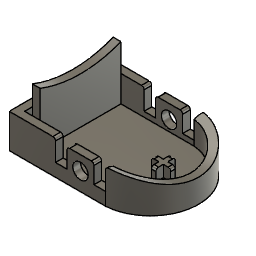
Vacuum_release_button (Autodesk Fusion 360 design; units mm, degrees)
Autodesk Fusion 360 part; units mm, degrees
sketch "Sketch1" plane through (0, 0, 0) normal (0, 1, 0) x (1, 0, 0)
  line L0 (-13.97, -9.525) -> (-13.97, 9.525)
  line L1 (-13.97, 9.525) -> (13.97, 9.525)
  line L2 (13.97, 9.525) -> (13.97, -9.525)
  line L3 (13.97, -9.525) -> (-13.97, 9.525) construction
  line L4 (-13.97, -9.525) -> (13.97, 9.525) construction
  line L5 (5.08, 9.525) -> (5.08, -9.525) construction
  line L6 (5.08, 0) -> (13.97, 0) construction
  arc A0 (5.08, -9.525) -> (5.08, 9.525) centre (4.4223, 0) ccw
  line L7 (-13.97, 9.525) -> (13.97, 9.525)
  arc A1 (5.08, -9.525) -> (5.08, 9.525) centre (4.4223, 0) ccw
  line L8 (13.97, -9.525) -> (-13.97, -9.525)
  line L9 (-13.97, -9.525) -> (-13.97, 9.525)
  line L10 (-12.446, 8.001) -> (5.08, 8.001)
  line L11 (5.08, -8.001) -> (-12.446, -8.001)
  line L12 (-12.446, -8.001) -> (-12.446, 8.001)
  line L13 (13.97, 0) -> (12.446, 0) construction
  arc A2 (5.08, -8.001) -> (5.08, 8.001) centre (4.4176, 0) ccw
  line L14 (-10.922, 8.001) -> (-10.922, -8.001)
  line L15 (-9.398, 8.001) -> (-9.398, -8.001)
  line L16 (2.794, 9.525) -> (2.794, 8.001)
  line L17 (2.794, -8.001) -> (2.794, -9.525)
  line L18 (-2.54, 9.525) -> (-2.54, 8.001)
  line L19 (-2.54, -8.001) -> (-2.54, -9.525)
  line L20 (-4.826, 9.525) -> (-4.826, 8.001)
  line L21 (-4.826, -8.001) -> (-4.826, -9.525)
  line L22 (5.08, 9.525) -> (5.08, 8.001)
  line L23 (5.08, -8.001) -> (5.08, -9.525)
  line L24 (5.08, 0.4445) -> (8.89, 0.4445)
  line L25 (8.89, 0.4445) -> (8.89, -0.4445)
  line L26 (8.89, -0.4445) -> (5.08, -0.4445)
  line L27 (5.08, -0.4445) -> (5.08, 0.4445)
  line L28 (5.08, 0) -> (6.985, 0) construction
  line L29 (7.4295, 1.905) -> (6.5405, 1.905)
  line L30 (6.5405, 1.905) -> (6.5405, -1.905)
  line L31 (6.5405, -1.905) -> (7.4295, -1.905)
  line L32 (7.4295, -1.905) -> (7.4295, 1.905)
  line L33 (7.4295, 1.905) -> (6.5405, -1.905) construction
  line L34 (6.5405, 1.905) -> (7.4295, -1.905) construction
  point P0 (6.985, 0)
  dimension "d2" = 19.05
  dimension "d4" = 9.525
  dimension "d5" = 9.525
  dimension "d6" = 27.94
  dimension "d7" = 19.05
  dimension "d12" = 1.524
  dimension "d13" = 1.524
  dimension "d14" = 1.524
  dimension "d17" = 19.05
  dimension "d18" = 19.05
  dimension "d19" = 1.524
  dimension "d20" = 1.524
  dimension "d21" = 1.524
  dimension "d22" = 16.764
  dimension "d23" = 11.43
  dimension "d24" = 16.764
  dimension "d25" = 11.43
  dimension "d26" = 2.286
  dimension "d27" = 2.286
  dimension "d38" = 3.81
  dimension "d39" = 0.889
  dimension "d40" = 0.4445
  dimension "d41" = 1.905
  dimension "d42" = 0.889
  dimension "d43" = 3.81
  constraint parallel L0 L2
  constraint coincident L3 origin
  constraint coincident L4 origin
  constraint coincident L1 L5.start
  constraint coincident L6.end A0
  constraint tangent L2 A0
  constraint horizontal L8
  constraint perpendicular L8 L9
  constraint parallel L7 L8
  constraint coincident L5.start L7
  constraint coincident L5.end L8
  constraint horizontal L11
  constraint perpendicular L11 L12
  constraint parallel L10 L11
  constraint perpendicular L2 L13
  constraint coincident L13.end A2
  constraint coincident L10 L14.start
  constraint coincident L11 L14.end
  constraint perpendicular L11 L14
  constraint coincident L10 L15.start
  constraint coincident L11 L15.end
  constraint perpendicular L11 L15
  constraint coincident L7 L16.start
  constraint coincident L10 L16.end
  constraint perpendicular L10 L16
  constraint coincident L11 L17.start
  constraint coincident L1 L18.start
  constraint coincident L10 L18.end
  constraint perpendicular L10 L18
  constraint coincident L11 L19.start
  constraint coincident L1 L20.start
  constraint coincident L10 L20.end
  constraint perpendicular L10 L20
  constraint coincident L11 L21.start
  constraint coincident L8 L21.end
  constraint perpendicular L8 L21
  constraint perpendicular L10 L22
  constraint perpendicular L8 L23
  constraint horizontal L24
  constraint vertical L25
  constraint horizontal L26
  constraint vertical L27
  constraint coincident L5 L24.start
  constraint coincident L6 P0
  constraint perpendicular L5 L28
  constraint horizontal L29
  constraint perpendicular L29 L30
  constraint parallel L29 L31
  constraint parallel L30 L32
  constraint coincident L33 P0
  constraint coincident L34 P0
  constraint coincident P0 L28.end
  measures "d2" distance of L0.start L0.end
  measures "d4" distance of L1.end L6.end
  measures "d5" distance of L2.end L6.end
  measures "d6" distance of L0.end L1.end
  measures "d7" distance of L0.start L0.end
  measures "d12" vertical distance of L0.end L10.start
  measures "d13" horizontal distance of L0.end L10.start
  measures "d14" vertical distance of L0.start L11.end
  measures "d17" horizontal distance of L0.start L11.start
  measures "d18" horizontal distance of L0.end L10.end
  measures "d19" distance of L6.end L13.end
  measures "d20" distance of L10.start L14.start
  measures "d21" distance of L14.start L15.start
  measures "d22" distance of L0.end L16.start
  measures "d23" distance of L0.end L18.start
  measures "d24" distance of L0.start L17.end
  measures "d25" distance of L0.start L19.end
  measures "d26" distance of L18.end L20.end
  measures "d27" distance of L19.end L21.end
  measures "d38" distance of L24.start L24.end
  measures "d39" distance of L24.start L26.end
  measures "d40" distance of L6.start L24.start
  measures "d41" distance of L6.start P0
  measures "d42" distance of L30.end L31.end
  measures "d43" distance of L29.end L30.end
extrude "Extrude1" add sketch "Sketch1" along normal blind 6.731 contours L0 L1 L7 L8 L9 L10 L11 L12 L20 L21 | A0 A1 A2 L22 L23 makes body 1 at (9.3779, 4.4873, -8.1609) makes body 2 at (-13.97, 4.4873, 3.175)
extrude "Extrude2" add sketch "Sketch1" along normal blind 12.192 contours L10 L11 L14 L15 bodies 2
extrude "Extrude3" add sketch "Sketch1" along normal blind 1.524 contours L10 L11 A2 L15 | L10 L11 L12 L14 | L24 L26 L27 L30 | L24 L29 L30 L32 | L24 L26 L30 L32 | L24 L25 L26 L32 | L26 L30 L31 L32 bodies 1 2
extrude "Extrude4" add sketch "Sketch1" along normal blind 2.54 contours L8 L11 L19 L21 | L1 L7 L10 L18 L20 | L8 L11 L17 L23 | L1 L7 L10 L16 L22 bodies 1
extrude "Extrude5" add sketch "Sketch1" along normal blind 6.35 contours L8 L11 L17 L19 | L1 L7 L10 L16 L18 bodies 1
extrude "Extrude6" add sketch "Sketch1" along normal blind 3.81 contours L24 L26 L27 L30 | L24 L29 L30 L32 | L24 L26 L30 L32 | L24 L25 L26 L32 | L26 L30 L31 L32 bodies 1
sketch "Sketch2" plane through (-10.922, 0, 0) normal (-1, 0, 0) x (0, 0, 1)
  line L0 (-8.001, 1.524) -> (8.001, 1.524)
  line L1 (8.001, 1.524) -> (8.001, 6.731)
  line L2 (8.001, 6.731) -> (8.001, 12.192)
  line L3 (8.001, 12.192) -> (-8.001, 12.192)
  line L4 (-8.001, 12.192) -> (-8.001, 6.731)
  line L5 (-8.001, 6.731) -> (-8.001, 1.524)
  line L6 (0, 12.192) -> (0, 10.668)
  arc A0 (-8.001, 12.192) -> (8.001, 12.192) centre (0, 32.4326) ccw
  dimension "d46" = 1.524
  constraint midpoint L3 L6.start
  constraint perpendicular L3 L6
  constraint coincident L6.end A0
  constraint coincident L2.end L3.start
  constraint coincident L3.end L4.start
  measures "d46" distance of L6.start L6.end
extrude "Extrude7" cut sketch "Sketch2" against normal up to surface (1.524 mm away) contours L3 L6 A0 | L3 L6 A0 bodies 1
sketch "Sketch3" plane through (0, 0, -9.525) normal (0, 0, -1) x (-1, 0, 0)
  line L0 (-5.08, 0) -> (13.97, 0)
  line L1 (13.97, 0) -> (13.97, 6.731)
  line L2 (13.97, 6.731) -> (4.826, 6.731)
  line L3 (4.826, 6.731) -> (4.826, 2.54)
  line L4 (4.826, 2.54) -> (2.54, 2.54)
  line L5 (2.54, 2.54) -> (2.54, 6.35)
  line L6 (2.54, 6.35) -> (-2.794, 6.35)
  line L7 (-2.794, 6.35) -> (-2.794, 2.54)
  line L8 (-2.794, 2.54) -> (-5.08, 2.54)
  line L9 (-5.08, 2.54) -> (-5.08, 0)
  line L10 (-2.794, 3.556) -> (2.54, 3.556) construction
  line L11 (-0.127, 6.35) -> (-0.127, 3.556) construction
  circle A0 centre (-0.127, 3.556) radius 1.524
  dimension "d49" = 2.667
  dimension "d50" = 2.794
  dimension "d51" = 3.048
  constraint coincident L7 L10.start
  constraint coincident L5 L10.end
  constraint perpendicular L5 L10
  constraint coincident L6 L11.start
  constraint coincident L10 L11.end
  constraint perpendicular L10 L11
  constraint coincident L11.end A0.centre
  measures "d49" distance of L6.end L11.start
  measures "d50" distance of L6.end L10.start
  measures "d51" diameter of A0
extrude "Extrude8" cut sketch "Sketch3" against normal up to surface (19.05 mm away) contours A0 bodies 1
fillet "Fillet1" radius 0.508 12 edges at (-4.826, 6.731, -8.763) (-2.54, 6.35, -8.763) (2.794, 6.35, -8.763) (5.08, 6.731, -8.763) (5.08, 6.731, 8.763) (2.794, 6.35, 8.763) (-2.54, 6.35, 8.763) (-4.826, 6.731, 8.763) (5.08, 3.81, 0) (6.985, 3.81, -1.905) (6.985, 3.81, 1.905) (8.89, 3.81, 0) on bodies 1
ref_plane "WorkPlane2" through (5.08, 3.3655, 0) normal (-1, 0, 0) x (0, 0, 1)
sketch "Sketch6" plane through (5.08, 3.3655, 0) normal (-1, 0, 0) x (0, 0, -1)
  line L0 (9.524, -3.3789) -> (-9.526, -3.3789)
  arc A0 (9.524, -3.3789) -> (-9.526, -3.3789) centre (-0.001, -23.9778) ccw
  dimension "d58" = 19.05
  constraint horizontal L0
  measures "d58" distance of L0.start L0.end
extrude "Extrude9" cut sketch "Sketch6" against normal blind 8.89 bodies 1
named bodies: "Vacuum_Release_Button"
